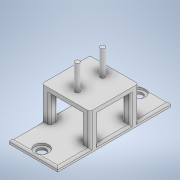
# Autodesk Inventor part: uv-vis cell holder_pins
Saved by Autodesk Inventor 2020 (Build 240168000, 168)
## iProperties
Created: 2023-03-31
Part Number: uv-vis cell holder_pins
Material: Generic
Document SubType Name: Modeling
Designer: Beaucage
Density: 1 g/cm^3
Appearance: Default
Author: Beaucage
Autodesk Inventor part; units mm, degrees
ref_plane "YZ Plane" through (0, 0, 0) normal (1, 0, 0) x (0, 1, 0)
ref_plane "XZ Plane" through (0, 0, 0) normal (0, 1, 0) x (-1, 0, 0)
ref_plane "XY Plane" through (0, 0, 0) normal (0, 0, 1) x (1, 0, 0)
sketch "Sketch2" plane through (0, 0, 0) normal (0, 1, 0) x (-1, 0, 0)
  line L0 (0, 0) -> (38.1, 0)
  line L1 (38.1, 0) -> (38.1, -38.1)
  line L2 (38.1, -38.1) -> (0, -38.1)
  line L3 (0, -38.1) -> (0, 0)
  dimension "d0" = 38.1
  dimension "d1" = 38.1
  constraints: 8 end point, 2 parallel, 1 horizontal, 1 perpendicular
  measures "d0" distance of L1.end L2.end
  measures "d1" distance of L0.end L1.end
extrude "Extrusion1" add sketch "Sketch2" along normal blind 3.175
sketch "Sketch3" plane through (0, 3.175, 0) normal (0, 1, 0) x (1, 0, 0)
  line L0 (-38.1, 38.1) -> (-38.1, 0) projected
  line L1 (-38.1, 19.05) -> (-19.05, 19.05)
  line L2 (-19.05, 19.05) -> (-19.05, 29.05)
  line L3 (-19.05, 29.05) -> (-19.05, 9.05)
  circle A0 centre (-19.05, 9.05) radius 1.8
  circle A1 centre (-19.05, 29.05) radius 1.8
  point P0 (0, 0)
  dimension "d4" = 19.05
  dimension "d5" = 10
  dimension "d6" = 20
  dimension "d41" = 3.6
  dimension "d42" = 3.6
  constraints: 6 end point, 2 centre point, 2 coincident, 1 horizontal, 1 midpoint, 1 perpendicular, 1 point on line
  measures "d4" distance of L1.start L1.end
  measures "d5" distance of L1.end L2.end
  measures "d6" distance of L2.end L3.end
  measures "d41" diameter of A0
  measures "d42" diameter of A1
sketch "Sketch4" plane through (0, 0, 0) normal (0, -1, 0) x (1, 0, 0)
  line L0 (-38.1, 0) -> (0, 0) projected
  line L1 (0, 0) -> (-6.35, 0)
  line L2 (-6.35, 0) -> (-6.35, -6.35)
  line L3 (-6.35, -6.35) -> (0, -6.35)
  line L4 (0, -6.35) -> (0, 0)
  line L5 (0, 0) -> (0, -38.1) projected
  line L6 (0, -38.1) -> (-6.35, -38.1)
  line L7 (-6.35, -38.1) -> (-6.35, -31.75)
  line L8 (-6.35, -31.75) -> (0, -31.75)
  line L9 (0, -31.75) -> (0, -38.1)
  line L10 (0, -38.1) -> (-38.1, -38.1) projected
  line L11 (-38.1, -38.1) -> (-31.75, -38.1)
  line L12 (-31.75, -38.1) -> (-31.75, -31.75)
  line L13 (-31.75, -31.75) -> (-38.1, -31.75)
  line L14 (-38.1, -31.75) -> (-38.1, -38.1)
  line L15 (-38.1, -38.1) -> (-38.1, 0) projected
  line L16 (-38.1, 0) -> (-31.75, 0)
  line L17 (-31.75, 0) -> (-31.75, -6.35)
  line L18 (-31.75, -6.35) -> (-38.1, -6.35)
  line L19 (-38.1, -6.35) -> (-38.1, 0)
  dimension "d14" = 6.35
  dimension "d15" = 6.35
  dimension "d16" = 6.35
  dimension "d17" = 6.35
  dimension "d18" = 6.35
  dimension "d19" = 6.35
  dimension "d20" = 6.35
  dimension "d21" = 6.35
  constraints: 32 end point, 8 parallel, 4 horizontal, 4 perpendicular
  measures "d14" distance of L3.end L2.end
  measures "d15" distance of L2.end L1.end
  measures "d16" distance of L7.end L8.end
  measures "d17" distance of L6.end L7.end
  measures "d18" distance of L13.end L12.end
  measures "d19" distance of L12.end L11.end
  measures "d20" distance of L17.end L18.end
  measures "d21" distance of L16.end L17.end
extrude "Extrusion2" add sketch "Sketch4" along normal blind 25.4 contours L0 L17 L18 L15 | L0 L4 L3 L2 | L13 L12 L10 L14 | L5 L6 L7 L8
sketch "Sketch5" plane through (0, -25.4, 0) normal (0, -1, 0) x (1, 0, 0)
  line L0 (0, 0) -> (-38.1, 0)
  line L1 (-38.1, 0) -> (-38.1, -63.5)
  line L2 (-38.1, -63.5) -> (0, -63.5)
  line L3 (0, -63.5) -> (0, 0)
  line L4 (0, 0) -> (-38.1, 0)
  line L5 (-38.1, 0) -> (-38.1, 25.4)
  line L6 (-38.1, 25.4) -> (0, 25.4)
  line L7 (0, 25.4) -> (0, 0)
  dimension "d24" = 38.1
  dimension "d25" = 63.5
  dimension "d26" = 25.4
  constraints: 16 end point, 4 parallel, 2 horizontal, 2 perpendicular, 1 point on line
  measures "d24" distance of L2.end L1.end
  measures "d25" distance of L1.end L0.end
  measures "d26" distance of L4.end L5.end
extrude "Extrusion3" add sketch "Sketch5" against normal blind 3.175
sketch "Sketch6" plane through (0, -22.225, 0) normal (0, 1, 0) x (1, 0, 0)
  line L0 (-38.1, -25.4) -> (-38.1, 63.5) projected
  line L1 (-38.1, -25.4) -> (-38.1, 19.05)
  line L2 (-38.1, 19.05) -> (-19.05, 19.05)
  line L3 (-19.05, 19.05) -> (-19.05, 57.15)
  line L4 (-19.05, 57.15) -> (-19.05, -19.05)
  point P0 (0, 0)
  dimension "d29" = 44.45
  dimension "d30" = 19.05
  dimension "d31" = 38.1
  dimension "d32" = 76.2
  constraints: 8 end point, 2 perpendicular, 1 midpoint, 1 point on line
  measures "d29" distance of L0.start L1.end
  measures "d30" distance of L1.end L2.end
  measures "d31" distance of L2.end L3.end
  measures "d32" distance of L3.end L4.end
hole "Hole2" at (-19.05, -22.225, 19.05) at (-19.05, -22.225, -57.15) direction (0, -1, 0) diameter 6.7564 depth 11.4875 counterbore diameter 11.1252 counterbore depth 1.5875 clearance for "Socket Head Cap Screw" size "1/4" standard "Ansi Unified Screw Threads"
fillet "Fillet1" radius 1.5875 24 edges at (-38.1, -9.525, 0) (-31.75, -11.1125, 0) (0, -9.525, 0) (-6.35, -11.1125, 0) (0, -11.1125, -6.35) (0, -11.1125, -31.75) (0, -9.525, -38.1) (0, -22.225, -50.8) (0, -22.225, -19.05) (0, -22.225, 12.7) (-19.05, -22.225, 25.4) (-38.1, -22.225, 12.7) (-19.05, -22.225, -63.5) (-38.1, -22.225, -50.8) (-31.75, -11.1125, -38.1) (-6.35, -11.1125, -38.1) (-38.1, -9.525, -38.1) (-38.1, -22.225, -19.05) (-38.1, -11.1125, -6.35) (-38.1, -11.1125, -31.75) (-31.75, -11.1125, -6.35) (-6.35, -11.1125, -31.75) (-6.35, -11.1125, -6.35) (-31.75, -11.1125, -31.75)
extrude "Extrusion4" add sketch "Sketch3" along normal blind 20
body "Solid1"
